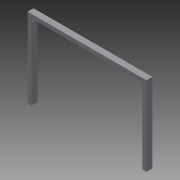
# Autodesk Inventor part: base extend
Saved by Autodesk Inventor 2015 (Build 190159000, 159)
## iProperties
Created: 2016-05-27
Part Number: base extend
Material: Generic
Document SubType Name: Modeling
Designer: Toby
Density: 1 g/cm^3
Appearance: Default
Author: Toby
Autodesk Inventor part; units mm, degrees
ref_plane "YZ Plane" through (0, 0, 0) normal (1, 0, 0) x (0, 1, 0)
ref_plane "XZ Plane" through (0, 0, 0) normal (0, 1, 0) x (-1, 0, 0)
ref_plane "XY Plane" through (0, 0, 0) normal (0, 0, 1) x (1, 0, 0)
sketch "Sketch1" plane through (0, 0, 0) normal (0, 1, 0) x (-1, 0, 0)
  line L0 (27.5, 19.0625) -> (-32.5, 19.0625)
  line L1 (-32.5, 19.0625) -> (-32.5, 17.0625)
  line L2 (-32.5, 17.0625) -> (27.5, 17.0625)
  line L3 (27.5, 17.0625) -> (27.5, 19.0625)
  line L4 (27.5, 19.0625) -> (25.5, 19.0625)
  line L5 (25.5, 19.0625) -> (25.5, -20.9375)
  line L6 (25.5, -20.9375) -> (27.5, -20.9375)
  line L7 (27.5, -20.9375) -> (27.5, 19.0625)
  line L8 (-32.5, 19.0625) -> (-30.5, 19.0625)
  line L9 (-30.5, 19.0625) -> (-30.5, -20.9375)
  line L10 (-30.5, -20.9375) -> (-32.5, -20.9375)
  line L11 (-32.5, -20.9375) -> (-32.5, 19.0625)
  point P0 (0, 0)
  dimension "d0" = 2
  dimension "d1" = 0
  dimension "d2" = 2
  dimension "d3" = 2
  dimension "d4" = 60
  dimension "d5" = 40
  dimension "d6" = 40
  constraints: 24 end point, 6 parallel, 3 horizontal, 3 perpendicular, 2 point on line
  measures "d0" distance between parallel lines of L7 L5
  measures "d1" distance between parallel lines of L3 L7
  measures "d2" distance between parallel lines of L11 L9
  measures "d3" distance between parallel lines of L0 L2
  measures "d4" distance of L0.start L0.end
  measures "d5" distance of L4.end L5.end
  measures "d6" distance of L10.end L0.end
extrude "Extrusion1" add sketch "Sketch1" along normal blind 3
fillet "Fillet1" radius 2 2 edges at (-25.5, 1.5, 17.0625) (30.5, 1.5, 17.0625)
body "Solid1"
